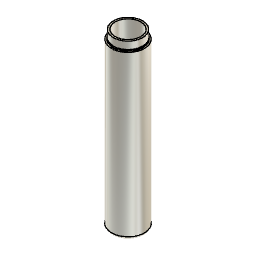
Cesaroni 29Pro 2G casing v3 (Autodesk Fusion 360 design; units mm, degrees)
Autodesk Fusion 360 part; units mm, degrees
sketch "Sketch1" plane through (0, 0, 0) normal (0, 0, 1) x (1, 0, 0)
  circle A0 centre (0, 0) radius 14.2875
  dimension "d1" = 28.575
  constraint coincident A0.centre origin
  measures "d1" diameter of A0
extrude "Extrude1" add sketch "Sketch1" along normal blind 142.24 thin wall 3.175 on the right open curves A0
extrude "Extrude2" add sketch "Sketch1" along normal blind 3.175
fillet "Fillet1" radius 2.5 1 edges at (-13.3206, -5.1666, 0)
sketch "Sketch2" plane through (0, 0, 142.24) normal (0, 0, 1) x (-1, 0, 0)
  circle A0 centre (0, 0) radius 11.1125
  circle A1 centre (0, 0) radius 14.2875
  circle A2 centre (0, 0) radius 12.7
  dimension "d15" = 25.4
  constraint coincident A0.centre A1.centre
  measures "d15" diameter of A2
extrude "Extrude3" add sketch "Sketch2" along normal mid plane 12.7 contours A2
sketch "Sketch3" plane through (0, 0, 142.24) normal (0, 0, 1) x (-1, 0, 0)
  circle A0 centre (0, 0) radius 14.2875
  circle A1 centre (0, 0) radius 12.7
  circle A2 centre (0, 0) radius 13
  dimension "d17" = 0.3
extrude "Extrude4" cut sketch "Sketch3" against normal blind 1 contours A0
sketch "Sketch4" plane through (0, 0, 0) normal (0, 0, -1) x (1, 0, 0)
  circle A0 centre (0, 0) radius 11.7875
  circle A1 centre (0, 0) radius 10
  dimension "d18" = 20
  constraint coincident A0.centre A1.centre
  measures "d18" diameter of A1
extrude "Extrude5" cut sketch "Sketch4" against normal blind 10 contours A1
